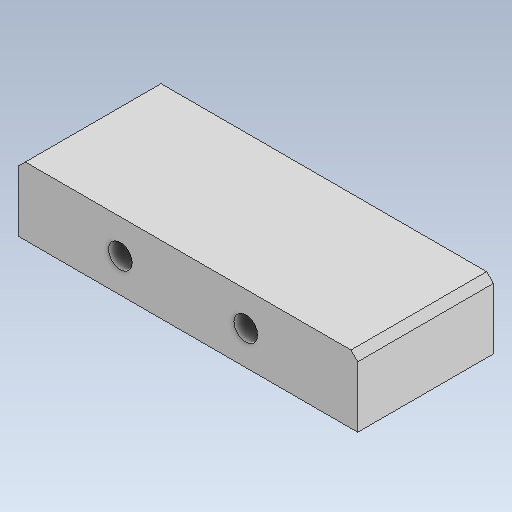
# Autodesk Inventor part: 10-06-013 Suport cutie
Saved by Autodesk Inventor 2020 (Build 240168000, 168)
## iProperties
Created: 2019-12-30
Part Number: 10-06-013 Suport cutie
Material: Generic
Document SubType Name: Modeling
Designer: iuliu
Density: 1 g/cm^3
Appearance: Default
Description: Suport cutie Arduino
Mass: 76.7612 g
Surface Area: 151.036 cm^2
Volume: 76.7612 cm^3
Author: iuliu
Subject: 026
Autodesk Inventor part; units mm, degrees
ref_plane "YZ Plane" through (0, 0, 0) normal (1, 0, 0) x (0, 1, 0)
ref_plane "XZ Plane" through (0, 0, 0) normal (0, 1, 0) x (-1, 0, 0)
ref_plane "XY Plane" through (0, 0, 0) normal (0, 0, 1) x (1, 0, 0)
sketch "Sketch1" plane through (0, 0, 0) normal (0, 0, 1) x (1, 0, 0)
  line L0 (-50, 10) -> (50, 10)
  line L1 (50, 10) -> (50, -10)
  line L2 (50, -10) -> (-50, -10)
  line L3 (-50, -10) -> (-50, 10)
  circle A0 centre (-20, 0) radius 3.5
  circle A1 centre (17, 0) radius 3.5
  point P0 (0, 0)
  point P1 (0, 10)
  point P2 (-50, 0)
  dimension "d0" = 20
  dimension "d1" = 100
  dimension "d2" = 10
  dimension "d3" = 30
  dimension "d4" = 33
  dimension "d5" = 7
  dimension "d6" = 7
  constraints: 8 end point, 2 centre point, 2 coincident, 2 horizontal alignment, 2 midpoint, 2 parallel, 1 horizontal, 1 perpendicular, 1 vertical alignment
  measures "d0" distance of L2.end L0.start
  measures "d1" distance of L0.start L0.end
  measures "d2" distance from line of point (-20, 0) L0
  measures "d3" distance from line of L3 point (-20, 0)
  measures "d4" distance from line of point (17, 0) L1
  measures "d5" diameter of A0
  measures "d6" diameter of A1
extrude "Extrusion1" add sketch "Sketch1" along normal blind 40
chamfer "Chamfer1" distance 2 angle 45 2 edges at (-50, 10, 20) (50, 10, 20)
body "Solid1"
